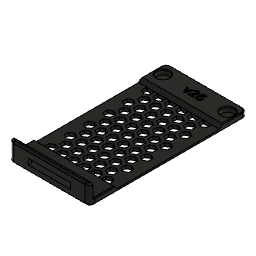
Door_Mount_M1 (Autodesk Fusion 360 design; units mm, degrees)
Autodesk Fusion 360 part; units mm, degrees
note: some values were not read from the file. Set by a fixed rule: which sketch regions a step uses.
(part 1 of 2)
sketch "Skizze1" plane through (0, 0, 0) normal (0, 0, 1) x (1, 0, 0)
  line L0 (22, -48.5) -> (-22, -48.5)
  line L1 (-25, -45.5) -> (-25, 45.5)
  line L2 (-22, 48.5) -> (22, 48.5)
  line L3 (25, 45.5) -> (25, -45.5)
  line L4 (25, -48.5) -> (-25, 48.5) construction
  line L5 (-25, -48.5) -> (25, 48.5) construction
  arc A0 (-22, 48.5) -> (-25, 45.5) centre (-22, 45.5) ccw
  arc A1 (25, 45.5) -> (22, 48.5) centre (22, 45.5) ccw
  arc A2 (22, -48.5) -> (25, -45.5) centre (22, -45.5) ccw
  arc A3 (-25, -45.5) -> (-22, -48.5) centre (-22, -45.5) ccw
  dimension "d356" = 50
  dimension "d357" = 97
  dimension "d358" = 3
  constraint horizontal L0
  constraint perpendicular L0 L1
  constraint parallel L0 L2
  constraint parallel L1 L3
  constraint coincident L4 origin
  constraint coincident L5 origin
  constraint coincident L4.end L1
  constraint coincident L4.end L2
  constraint tangent L1 A0
  constraint tangent L2 A0
  constraint coincident L5.end L2
  constraint coincident L5.end L3
  constraint tangent L2 A1
  constraint tangent L3 A1
  constraint equal A0 A1
  constraint coincident L4.start L3
  constraint coincident L4.start L0
  constraint tangent L3 A2
  constraint tangent L0 A2
  constraint equal A0 A2
  constraint coincident L5.start L0
  constraint coincident L5.start L1
  constraint tangent L0 A3
  constraint tangent L1 A3
  constraint equal A0 A3
  measures "d356" distance of L4.end L5.end
  measures "d357" distance of L5.start L4.end
  measures "d358" radius of A0
extrude "Extrusion1" add sketch "Skizze1" along normal blind 4
sketch "Skizze2" plane through (0, 0, 4) normal (0, 0, 1) x (-1, 0, 0)
  line L0 (24.8284, 46.5) -> (-24.8284, 46.5)
  line L1 (22, 48.5) -> (-22, 48.5)
  arc A0 (-22, 48.5) -> (-25, 45.5) centre (-22, 45.5) ccw
  arc A1 (25, 45.5) -> (22, 48.5) centre (22, 45.5) ccw
  dimension "d416" = 2
  constraint horizontal L0
  constraint coincident L0.end A0
  constraint coincident L0.start A1
  measures "d416" distance of L0 L1
extrude "Extrusion2" add sketch "Skizze2" along normal blind 8
ref_plane "Arbeitsebene1" through (0, 0, 4) normal (0, 0, 1) x (1, 0, 0)
sketch "Skizze3" plane through (0, 0, 4) normal (0, 0, 1) x (1, 0, 0)
  line L0 (-22, -48.5) -> (22, -48.5)
  line L1 (22, -48.5) -> (-22, -48.5)
  line L2 (-13, -46.5) -> (13, -46.5)
  line L3 (13, -46.5) -> (13, -48.5)
  line L4 (13, -48.5) -> (-13, -48.5)
  line L5 (-13, -48.5) -> (-13, -46.5)
  line L6 (-22, 48.5) -> (22, 48.5)
  line L7 (24.8284, -46.5) -> (-24.8284, -46.5)
  dimension "d371" = 26
  dimension "d372" = 13
  constraint horizontal L2
  constraint vertical L3
  constraint horizontal L4
  constraint vertical L5
  constraint coincident L0 L3.end
  constraint coincident L2.start L7
  measures "d371" distance of L3 L5
  measures "d372" distance of origin L5
extrude "Extrusion3" cut sketch "Skizze3" along normal blind 3.5
sketch "Skizze5" plane through (0, 0, 4) normal (0, 0, 1) x (-1, 0, 0)
  line L0 (-25, 45.5) -> (-25, -45.5)
  arc A0 (-25, -45.5) -> (-22, -48.5) centre (-22, -45.5) ccw
  line L1 (-22, -48.5) -> (22, -48.5)
  arc A1 (22, -48.5) -> (25, -45.5) centre (22, -45.5) ccw
  line L2 (25, -45.5) -> (25, 45.5)
  circle A2 centre (20, -41.5) radius 3.75
  circle A3 centre (-20, -41.5) radius 3.75
  line L3 (24.8284, 46.5) -> (13, 46.5)
  arc A4 (-24.8284, 46.5) -> (-25, 45.5) centre (-22, 45.5) ccw
  arc A5 (25, 45.5) -> (24.8284, 46.5) centre (22, 45.5) ccw
  line L4 (13, 46.5) -> (13, 48.5)
  line L5 (13, 48.5) -> (-13, 48.5)
  line L6 (-13, 48.5) -> (-13, 46.5)
  line L7 (-13, 46.5) -> (-24.8284, 46.5)
  dimension "d406" = 7.5
  dimension "d407" = 40
  dimension "d408" = 20
  constraint horizontal A2.centre A3.centre
  constraint equal A2 A3
  measures "d406" diameter of A2
  measures "d407" distance of A2.centre A3.centre
  measures "d408" horizontal distance of origin A2.centre
extrude "Extrusion4" cut sketch "Skizze5" against normal blind 3 contours A2 | A3
sketch "Skizze6" plane through (0, 0, 4) normal (0, 0, 1) x (-1, 0, 0)
  line L0 (24.8284, 46.5) -> (13, 46.5)
  line L1 (13, 46.5) -> (13, 48.5)
  line L2 (13, 48.5) -> (-13, 48.5)
  line L3 (-13, 48.5) -> (-13, 46.5)
  line L4 (-13, 46.5) -> (-24.8284, 46.5)
  line L5 (5.5, -38.5) -> (-5.5, -38.5) construction
  line L6 (-5.5, -38.5) -> (-5.5, -43.5) construction
  line L7 (-5.5, -43.5) -> (5.5, -43.5) construction
  line L8 (5.5, -43.5) -> (5.5, -38.5) construction
  circle A0 centre (20, -41.5) radius 3.75
  circle A1 centre (-20, -41.5) radius 3.75
  arc A2 (-24.8284, 46.5) -> (-25, 45.5) centre (-22, 45.5) ccw
  line L9 (-25, 45.5) -> (-25, -45.5)
  arc A3 (-25, -45.5) -> (-22, -48.5) centre (-22, -45.5) ccw
  line L10 (-22, -48.5) -> (22, -48.5)
  arc A4 (22, -48.5) -> (25, -45.5) centre (22, -45.5) ccw
  line L11 (25, -45.5) -> (25, 45.5)
  arc A5 (25, 45.5) -> (24.8284, 46.5) centre (22, 45.5) ccw
  dimension "d417" = 5
  dimension "d418" = 5
  dimension "d420" = 11
  dimension "d435" = 5
  text T0 "v25" font "Arial" height 5 bold align centre middle in box 11 x 5 at (5.5, -38.5) x (-1, 0) y (0, -1) spacing 1
  constraint vertical origin
  measures "d435" distance of L7 L10
extrude "Extrusion5" cut sketch "Skizze6" against normal blind 0.3 text T0
sketch "Skizze8" plane through (0, 0, 4) normal (0, 0, 1) x (-1, 0, 0)
  line L0 (24.8284, 46.5) -> (13, 46.5)
  line L1 (13, 46.5) -> (13, 48.5)
  line L2 (13, 48.5) -> (-13, 48.5)
  line L3 (-13, 48.5) -> (-13, 46.5)
  line L4 (-13, 46.5) -> (-24.8284, 46.5)
  arc A0 (-24.8284, 46.5) -> (-25, 45.5) centre (-22, 45.5) ccw
  line L5 (-25, 45.5) -> (-25, -45.5)
  arc A1 (-25, -45.5) -> (-22, -48.5) centre (-22, -45.5) ccw
  line L6 (-22, -48.5) -> (22, -48.5)
  arc A2 (22, -48.5) -> (25, -45.5) centre (22, -45.5) ccw
  line L7 (25, -45.5) -> (25, 45.5)
  arc A3 (25, 45.5) -> (24.8284, 46.5) centre (22, 45.5) ccw
  circle A4 centre (-20, -41.5) radius 3.75
  circle A5 centre (20, -41.5) radius 3.75
  line L8 (1.9407, -42.1221) -> (3.3799, -38.5)
  line L9 (3.3799, -38.5) -> (4.2428, -38.5)
  line L10 (4.2428, -38.5) -> (5.7026, -42.1221)
  line L11 (5.7026, -42.1221) -> (4.6965, -42.1221)
  line L12 (4.6965, -42.1221) -> (4.0143, -40.2735)
  line L13 (4.0143, -40.2735) -> (3.8165, -39.6562)
  spline S0 degree 3 poles (3.8165, -39.6562) (3.7947, -39.7212) (3.7602, -39.8241) (3.7291, -39.9282) (3.7176, -39.9666) knots 0 0 0 0 0.020546 0.032577 0.032577 0.032577 0.032577
  spline S1 degree 3 poles (3.7176, -39.9666) (3.7014, -40.0178) (3.6688, -40.1207) (3.6332, -40.2225) (3.6153, -40.2735) knots 0 0 0 0 0.016125 0.032358 0.032358 0.032358 0.032358
  line L14 (3.6153, -40.2735) -> (2.9263, -42.1221)
  line L15 (2.9263, -42.1221) -> (1.9407, -42.1221)
  line L16 (-1.678, -39.3902) -> (-1.678, -38.5)
  line L17 (-1.678, -38.5) -> (1.6814, -38.5)
  spline S2 degree 3 poles (1.6814, -38.5) (1.6537, -38.6668) (1.5977, -39.0038) (1.4358, -39.3047) (1.354, -39.4567) knots 0 0 0 0 0.050353 0.101733 0.101733 0.101733 0.101733
  spline S3 degree 3 poles (0.2763, -40.6555) (0.0973, -40.8199) (-0.1834, -41.0777) (-0.4293, -41.3686) (-0.5184, -41.4741) knots 0 0 0 0 0.072782 0.114179 0.114179 0.114179 0.114179
  spline S4 degree 3 poles (-0.5184, -41.4741) (-0.5761, -41.5697) (-0.6853, -41.7511) (-0.7063, -41.9614) (-0.7162, -42.0607) knots 0 0 0 0 0.033023 0.0626 0.0626 0.0626 0.0626
  line L18 (25, -33.5) -> (-25, -33.5)
  line L19 (25, 33.5) -> (-25, 33.5)
  line L20 (-13, 48.5) -> (13, 48.5)
  line L21 (13, 48.5) -> (-13, 48.5)
  line L22 (22, 48.5) -> (-22, 48.5)
  line L23 (-22, 48.5) -> (22, 48.5)
  spline S5 degree 3 poles (1.5689, -42.0402) (1.5336, -42.2784) (1.469, -42.7135) (1.1692, -43.0319) (1.0334, -43.176) knots 0 0 0 0 0.070212 0.128259 0.128259 0.128259 0.128259
  spline S6 degree 3 poles (1.0334, -43.176) (0.8691, -43.2764) (0.5241, -43.4872) (0.1197, -43.509) (-0.0921, -43.5205) knots 0 0 0 0 0.056857 0.119356 0.119356 0.119356 0.119356
  spline S7 degree 3 poles (-0.0921, -43.5205) (-0.3201, -43.5088) (-0.7475, -43.4868) (-1.0936, -43.2377) (-1.2551, -43.1214) knots 0 0 0 0 0.06683 0.125293 0.125293 0.125293 0.125293
  spline S8 degree 3 poles (-1.678, -42.1289) (-1.6731, -42.0181) (-1.6634, -41.798) (-1.5923, -41.5895) (-1.557, -41.486) knots 0 0 0 0 0.033094 0.065719 0.065719 0.065719 0.065719
  spline S9 degree 3 poles (-1.557, -41.486) (-1.5082, -41.3799) (-1.4037, -41.1528) (-1.2534, -40.9529) (-1.1733, -40.8465) knots 0 0 0 0 0.034948 0.074768 0.074768 0.074768 0.074768
  spline S10 degree 3 poles (0.4093, -42.545) (0.4624, -42.4673) (0.5854, -42.2873) (0.6036, -42.0688) (0.6139, -41.9447) knots 0 0 0 0 0.027816 0.064377 0.064377 0.064377 0.064377
  spline S11 degree 3 poles (-1.2551, -43.1214) (-1.3785, -42.9797) (-1.6266, -42.6947) (-1.6608, -42.3182) (-1.678, -42.1289) knots 0 0 0 0 0.054863 0.110365 0.110365 0.110365 0.110365
  spline S12 degree 3 poles (-1.1733, -40.8465) (-1.0933, -40.7552) (-0.8965, -40.5305) (-0.6764, -40.3286) (-0.5457, -40.2087) knots 0 0 0 0 0.036404 0.089534 0.089534 0.089534 0.089534
  spline S13 degree 3 poles (-0.5457, -40.2087) (-0.4207, -40.0948) (-0.2242, -39.9158) (-0.0386, -39.7255) (0.029, -39.6562) knots 0 0 0 0 0.050705 0.079736 0.079736 0.079736 0.079736
  spline S14 degree 3 poles (0.029, -39.6562) (0.0667, -39.6122) (0.1387, -39.5283) (0.1973, -39.4347) (0.2251, -39.3902) knots 0 0 0 0 0.017365 0.033092 0.033092 0.033092 0.033092
  line L24 (0.2251, -39.3902) -> (-1.678, -39.3902)
  spline S15 degree 3 poles (1.354, -39.4567) (1.2231, -39.6357) (0.9046, -40.0712) (0.5091, -40.439) (0.2763, -40.6555) knots 0 0 0 0 0.066412 0.161523 0.161523 0.161523 0.161523
  spline S16 degree 3 poles (-0.7162, -42.0607) (-0.7115, -42.1588) (-0.7028, -42.3409) (-0.5942, -42.4864) (-0.544, -42.5535) knots 0 0 0 0 0.028676 0.053274 0.053274 0.053274 0.053274
  spline S17 degree 3 poles (-0.544, -42.5535) (-0.4783, -42.6037) (-0.3384, -42.7107) (-0.1619, -42.7205) (-0.0682, -42.7258) knots 0 0 0 0 0.024236 0.051648 0.051648 0.051648 0.051648
  spline S18 degree 3 poles (-0.0682, -42.7258) (0.0251, -42.7198) (0.2033, -42.7084) (0.3429, -42.5977) (0.4093, -42.545) knots 0 0 0 0 0.02732 0.052153 0.052153 0.052153 0.052153
  line L25 (0.6139, -41.9447) -> (1.5689, -42.0402)
  line L26 (-2.3397, -39.7858) -> (-3.2947, -39.8847)
  line L27 (-3.2333, -40.7169) -> (-2.4557, -40.8295)
  line L28 (-2.4557, -40.8295) -> (-2.9468, -43.4318)
  line L29 (-2.9468, -43.4318) -> (-5.4809, -43.4318)
  spline S19 degree 3 poles (-3.9905, -38.4147) (-3.7745, -38.4268) (-3.3639, -38.4497) (-3.0231, -38.6781) (-2.8615, -38.7865) knots 0 0 0 0 0.063525 0.120818 0.120818 0.120818 0.120818
  spline S20 degree 3 poles (-2.8615, -38.7865) (-2.7303, -38.9238) (-2.4604, -39.2062) (-2.3807, -39.5891) (-2.3397, -39.7858) knots 0 0 0 0 0.055809 0.114768 0.114768 0.114768 0.114768
  spline S21 degree 3 poles (-3.2947, -39.8847) (-3.3134, -39.7839) (-3.3491, -39.5912) (-3.4762, -39.4424) (-3.5368, -39.3714) knots 0 0 0 0 0.030142 0.057653 0.057653 0.057653 0.057653
  spline S22 degree 3 poles (-3.5368, -39.3714) (-3.6058, -39.3162) (-3.7419, -39.2073) (-3.9152, -39.1905) (-4.0007, -39.1821) knots 0 0 0 0 0.025896 0.051072 0.051072 0.051072 0.051072
  spline S23 degree 3 poles (-4.0007, -39.1821) (-4.0975, -39.193) (-4.2949, -39.2153) (-4.4367, -39.3549) (-4.5089, -39.426) knots 0 0 0 0 0.028374 0.057844 0.057844 0.057844 0.057844
  spline S24 degree 3 poles (-4.5089, -39.426) (-4.5693, -39.5253) (-4.706, -39.7497) (-4.713, -40.0138) (-4.7169, -40.161) knots 0 0 0 0 0.03432 0.077565 0.077565 0.077565 0.077565
  spline S25 degree 3 poles (-4.7169, -40.161) (-4.7127, -40.2994) (-4.7052, -40.5493) (-4.5706, -40.7584) (-4.5106, -40.8516) knots 0 0 0 0 0.040617 0.073292 0.073292 0.073292 0.073292
  spline S26 degree 3 poles (-4.5106, -40.8516) (-4.4356, -40.9188) (-4.2826, -41.0557) (-4.0778, -41.073) (-3.9734, -41.0819) knots 0 0 0 0 0.02936 0.059879 0.059879 0.059879 0.059879
  spline S27 degree 3 poles (-3.9734, -41.0819) (-3.837, -41.0639) (-3.5501, -41.0261) (-3.3423, -40.8233) (-3.2333, -40.7169) knots 0 0 0 0 0.040186 0.084518 0.084518 0.084518 0.084518
  line L30 (-5.4809, -43.4318) -> (-5.4809, -42.5348)
  line L31 (-5.4809, -42.5348) -> (-3.6733, -42.5348)
  line L32 (-3.6733, -42.5348) -> (-3.5232, -41.6855)
  spline S28 degree 3 poles (-3.5232, -41.6855) (-3.6296, -41.7323) (-3.8385, -41.8241) (-4.0663, -41.8387) (-4.178, -41.8458) knots 0 0 0 0 0.03456 0.067885 0.067885 0.067885 0.067885
  spline S29 degree 3 poles (-4.178, -41.8458) (-4.3827, -41.8264) (-4.7926, -41.7874) (-5.1035, -41.5173) (-5.2592, -41.382) knots 0 0 0 0 0.060049 0.120305 0.120305 0.120305 0.120305
  spline S30 degree 3 poles (-5.2592, -41.382) (-5.3885, -41.2113) (-5.6577, -40.8558) (-5.6872, -40.4099) (-5.7026, -40.178) knots 0 0 0 0 0.062815 0.130829 0.130829 0.130829 0.130829
  spline S31 degree 3 poles (-5.7026, -40.178) (-5.6881, -39.9783) (-5.6592, -39.5816) (-5.4489, -39.2441) (-5.3445, -39.0764) knots 0 0 0 0 0.059089 0.1174 0.1174 0.1174 0.1174
  spline S32 degree 3 poles (-5.3445, -39.0764) (-5.164, -38.8834) (-4.7972, -38.4914) (-4.2621, -38.4406) (-3.9905, -38.4147) knots 0 0 0 0 0.076512 0.155431 0.155431 0.155431 0.155431
  dimension "d436" = 15
  dimension "d437" = 15
  constraint coincident L7 L18.start
  constraint coincident L5 L18.end
  constraint perpendicular L5 L18
  constraint coincident L7 L19.start
  constraint coincident L5 L19.end
  constraint perpendicular L5 L19
  measures "d436" distance of L6 L18
  measures "d437" distance of L19 L23
extrude "Extrusion6" cut sketch "Skizze8" against normal blind 2 contours L5 L7 L18 L19
chamfer "Fase1" distance 1 angle 45 11 edges at (0, -48.5, 0) (-24.1213, -47.6213, 0) (-25, 0, 0) (-24.1213, 47.6213, 0) (0, 48.5, 0) (24.1213, 47.6213, 0) (25, 0, 0) (24.1213, -47.6213, 0) (0, -48.5, 12) (-23.7321, -47.9495, 12) (23.7321, -47.9495, 12)
chamfer "Fase1" distance 0.5 angle 45 11 edges at (-16.5038, 40.1439, 4) (23.4962, 40.1439, 4) (25, -39.5, 4) (24.9568, -46.0073, 4) (25, 39.5, 4) (24.1213, 47.6213, 4) (0, 48.5, 4) (-24.1213, 47.6213, 4) (-25, 39.5, 4) (-24.9568, -46.0073, 4) (-25, -39.5, 4)
chamfer "Fase1" distance 2 angle 45 2 edges at (0, 33.5, 2) (0, -33.5, 2)
sketch "Skizze9" plane through (0, 0, 2) normal (0, 0, 1) x (-1, 0, 0)
  line L0 (25, -31.5) -> (25, 31.5)
  line L1 (-25, 31.5) -> (-25, -31.5)
  line L2 (-2.5, -1.4434) -> (0, -2.8868)
  line L3 (0, -2.8868) -> (2.5, -1.4434)
  line L4 (2.5, -1.4434) -> (2.5, 1.4434)
  line L5 (2.5, 1.4434) -> (0, 2.8868)
  line L6 (0, 2.8868) -> (-2.5, 1.4434)
  line L7 (-2.5, 1.4434) -> (-2.5, -1.4434)
  line L8 (-6, 4.6188) -> (-3.5, 3.1754)
  line L9 (-3.5, 3.1754) -> (-1, 4.6188)
  line L10 (-1, 4.6188) -> (-1, 7.5056)
  line L11 (-1, 7.5056) -> (-3.5, 8.9489)
  line L12 (-3.5, 8.9489) -> (-6, 7.5056)
  line L13 (-6, 7.5056) -> (-6, 4.6188)
  line L14 (0, 2.8868) -> (-1, 4.6188) construction
  line L15 (-7, 2.8868) -> (-9.5, 1.4434)
  line L16 (-9.5, 1.4434) -> (-9.5, -1.4434)
  line L17 (-9.5, -1.4434) -> (-7, -2.8868)
  line L18 (-7, -2.8868) -> (-4.5, -1.4434)
  line L19 (-4.5, -1.4434) -> (-4.5, 1.4434)
  line L20 (-4.5, 1.4434) -> (-7, 2.8868)
  line L21 (-3.5, 3.1754) -> (-4.5, 1.4434) construction
  line L22 (1, 7.5056) -> (1, 4.6188)
  line L23 (1, 4.6188) -> (3.5, 3.1754)
  line L24 (3.5, 3.1754) -> (6, 4.6188)
  line L25 (6, 4.6188) -> (6, 7.5056)
  line L26 (6, 7.5056) -> (3.5, 8.9489)
  line L27 (3.5, 8.9489) -> (1, 7.5056)
  line L28 (2.5, 1.4434) -> (3.5, 3.1754) construction
  line L29 (-24.5, -32.8246) -> (-22, -31.3812)
  line L30 (-22, -31.3812) -> (-22, -28.4944)
  line L31 (-22, -28.4944) -> (-24.5, -27.0511)
  line L32 (-24.5, -27.0511) -> (-27, -28.4944)
  line L33 (-27, -28.4944) -> (-27, -31.3812)
  line L34 (-27, -31.3812) -> (-24.5, -32.8246)
  line L35 (-25.5, -34.5566) -> (-28, -33.1132)
  line L36 (-25.5, -37.4434) -> (-25.5, -34.5566)
  line L37 (-28, -38.8868) -> (-25.5, -37.4434)
  line L38 (-30.5, -37.4434) -> (-28, -38.8868)
  line L39 (-30.5, -34.5566) -> (-30.5, -37.4434)
  line L40 (-28, -33.1132) -> (-30.5, -34.5566)
  line L41 (-31.5, -32.8246) -> (-29, -31.3812)
  line L42 (-29, -31.3812) -> (-29, -28.4944)
  line L43 (-29, -28.4944) -> (-31.5, -27.0511)
  line L44 (-34, -31.3812) -> (-31.5, -32.8246)
  line L45 (-31.5, -27.0511) -> (-34, -28.4944)
  line L46 (-34, -28.4944) -> (-34, -31.3812)
  line L47 (-35, -33.1132) -> (-37.5, -34.5566)
  line L48 (-32.5, -34.5566) -> (-35, -33.1132)
  line L49 (-32.5, -37.4434) -> (-32.5, -34.5566)
  line L50 (-35, -38.8868) -> (-32.5, -37.4434)
  line L51 (-37.5, -37.4434) -> (-35, -38.8868)
  line L52 (-37.5, -34.5566) -> (-37.5, -37.4434)
  line L53 (-10.5, -32.8246) -> (-8, -31.3812)
  line L54 (-8, -31.3812) -> (-8, -28.4944)
  line L55 (-8, -28.4944) -> (-10.5, -27.0511)
  line L56 (-10.5, -27.0511) -> (-13, -28.4944)
  line L57 (-13, -28.4944) -> (-13, -31.3812)
  line L58 (-13, -31.3812) -> (-10.5, -32.8246)
  line L59 (-11.5, -34.5566) -> (-14, -33.1132)
  line L60 (-11.5, -37.4434) -> (-11.5, -34.5566)
  line L61 (-14, -38.8868) -> (-11.5, -37.4434)
  line L62 (-16.5, -37.4434) -> (-14, -38.8868)
  line L63 (-16.5, -34.5566) -> (-16.5, -37.4434)
  line L64 (-14, -33.1132) -> (-16.5, -34.5566)
  line L65 (-17.5, -32.8246) -> (-15, -31.3812)
  line L66 (-15, -31.3812) -> (-15, -28.4944)
  line L67 (-15, -28.4944) -> (-17.5, -27.0511)
  line L68 (-20, -31.3812) -> (-17.5, -32.8246)
  line L69 (-17.5, -27.0511) -> (-20, -28.4944)
  line L70 (-20, -28.4944) -> (-20, -31.3812)
  line L71 (-21, -33.1132) -> (-23.5, -34.5566)
  line L72 (-18.5, -34.5566) -> (-21, -33.1132)
  line L73 (-18.5, -37.4434) -> (-18.5, -34.5566)
  line L74 (-21, -38.8868) -> (-18.5, -37.4434)
  line L75 (-23.5, -37.4434) -> (-21, -38.8868)
  line L76 (-23.5, -34.5566) -> (-23.5, -37.4434)
  line L77 (3.5, -32.8246) -> (6, -31.3812)
  line L78 (6, -31.3812) -> (6, -28.4944)
  line L79 (6, -28.4944) -> (3.5, -27.0511)
  line L80 (3.5, -27.0511) -> (1, -28.4944)
  line L81 (1, -28.4944) -> (1, -31.3812)
  line L82 (1, -31.3812) -> (3.5, -32.8246)
  line L83 (2.5, -34.5566) -> (0, -33.1132)
  line L84 (2.5, -37.4434) -> (2.5, -34.5566)
  line L85 (0, -38.8868) -> (2.5, -37.4434)
  line L86 (-2.5, -37.4434) -> (0, -38.8868)
  line L87 (-2.5, -34.5566) -> (-2.5, -37.4434)
  line L88 (0, -33.1132) -> (-2.5, -34.5566)
  line L89 (-3.5, -32.8246) -> (-1, -31.3812)
  line L90 (-1, -31.3812) -> (-1, -28.4944)
  line L91 (-1, -28.4944) -> (-3.5, -27.0511)
  line L92 (-6, -31.3812) -> (-3.5, -32.8246)
  line L93 (-3.5, -27.0511) -> (-6, -28.4944)
  line L94 (-6, -28.4944) -> (-6, -31.3812)
  line L95 (-7, -33.1132) -> (-9.5, -34.5566)
  line L96 (-4.5, -34.5566) -> (-7, -33.1132)
  line L97 (-4.5, -37.4434) -> (-4.5, -34.5566)
  line L98 (-7, -38.8868) -> (-4.5, -37.4434)
  line L99 (-9.5, -37.4434) -> (-7, -38.8868)
  line L100 (-9.5, -34.5566) -> (-9.5, -37.4434)
  line L101 (17.5, -32.8246) -> (20, -31.3812)
  line L102 (20, -31.3812) -> (20, -28.4944)
  line L103 (20, -28.4944) -> (17.5, -27.0511)
  line L104 (17.5, -27.0511) -> (15, -28.4944)
  line L105 (15, -28.4944) -> (15, -31.3812)
  line L106 (15, -31.3812) -> (17.5, -32.8246)
  line L107 (16.5, -34.5566) -> (14, -33.1132)
  line L108 (16.5, -37.4434) -> (16.5, -34.5566)
  line L109 (14, -38.8868) -> (16.5, -37.4434)
  line L110 (11.5, -37.4434) -> (14, -38.8868)
  line L111 (11.5, -34.5566) -> (11.5, -37.4434)
  line L112 (14, -33.1132) -> (11.5, -34.5566)
  line L113 (10.5, -32.8246) -> (13, -31.3812)
  line L114 (13, -31.3812) -> (13, -28.4944)
  line L115 (13, -28.4944) -> (10.5, -27.0511)
  line L116 (8, -31.3812) -> (10.5, -32.8246)
  line L117 (10.5, -27.0511) -> (8, -28.4944)
  line L118 (8, -28.4944) -> (8, -31.3812)
  line L119 (7, -33.1132) -> (4.5, -34.5566)
  line L120 (9.5, -34.5566) -> (7, -33.1132)
  line L121 (9.5, -37.4434) -> (9.5, -34.5566)
  line L122 (7, -38.8868) -> (9.5, -37.4434)
  line L123 (4.5, -37.4434) -> (7, -38.8868)
  line L124 (4.5, -34.5566) -> (4.5, -37.4434)
  line L125 (31.5, -32.8246) -> (34, -31.3812)
  line L126 (34, -31.3812) -> (34, -28.4944)
  line L127 (34, -28.4944) -> (31.5, -27.0511)
  line L128 (31.5, -27.0511) -> (29, -28.4944)
  line L129 (29, -28.4944) -> (29, -31.3812)
  line L130 (29, -31.3812) -> (31.5, -32.8246)
  line L131 (30.5, -34.5566) -> (28, -33.1132)
  line L132 (30.5, -37.4434) -> (30.5, -34.5566)
  line L133 (28, -38.8868) -> (30.5, -37.4434)
  line L134 (25.5, -37.4434) -> (28, -38.8868)
  line L135 (25.5, -34.5566) -> (25.5, -37.4434)
  line L136 (28, -33.1132) -> (25.5, -34.5566)
  line L137 (24.5, -32.8246) -> (27, -31.3812)
  line L138 (27, -31.3812) -> (27, -28.4944)
  line L139 (27, -28.4944) -> (24.5, -27.0511)
  line L140 (22, -31.3812) -> (24.5, -32.8246)
  line L141 (24.5, -27.0511) -> (22, -28.4944)
  line L142 (22, -28.4944) -> (22, -31.3812)
  line L143 (21, -33.1132) -> (18.5, -34.5566)
  line L144 (23.5, -34.5566) -> (21, -33.1132)
  line L145 (23.5, -37.4434) -> (23.5, -34.5566)
  line L146 (21, -38.8868) -> (23.5, -37.4434)
  line L147 (18.5, -37.4434) -> (21, -38.8868)
  line L148 (18.5, -34.5566) -> (18.5, -37.4434)
  line L149 (-24.5, -20.8246) -> (-22, -19.3812)
  line L150 (-22, -19.3812) -> (-22, -16.4944)
  line L151 (-22, -16.4944) -> (-24.5, -15.0511)
  line L152 (-24.5, -15.0511) -> (-27, -16.4944)
  line L153 (-27, -16.4944) -> (-27, -19.3812)
  line L154 (-27, -19.3812) -> (-24.5, -20.8246)
  line L155 (-25.5, -22.5566) -> (-28, -21.1132)
  line L156 (-25.5, -25.4434) -> (-25.5, -22.5566)
  line L157 (-28, -26.8868) -> (-25.5, -25.4434)
  line L158 (-30.5, -25.4434) -> (-28, -26.8868)
  line L159 (-30.5, -22.5566) -> (-30.5, -25.4434)
  line L160 (-28, -21.1132) -> (-30.5, -22.5566)
  line L161 (-31.5, -20.8246) -> (-29, -19.3812)
  line L162 (-29, -19.3812) -> (-29, -16.4944)
  line L163 (-29, -16.4944) -> (-31.5, -15.0511)
  line L164 (-34, -19.3812) -> (-31.5, -20.8246)
  line L165 (-31.5, -15.0511) -> (-34, -16.4944)
  line L166 (-34, -16.4944) -> (-34, -19.3812)
  line L167 (-35, -21.1132) -> (-37.5, -22.5566)
  line L168 (-32.5, -22.5566) -> (-35, -21.1132)
  line L169 (-32.5, -25.4434) -> (-32.5, -22.5566)
  line L170 (-35, -26.8868) -> (-32.5, -25.4434)
  line L171 (-37.5, -25.4434) -> (-35, -26.8868)
  line L172 (-37.5, -22.5566) -> (-37.5, -25.4434)
  line L173 (-10.5, -20.8246) -> (-8, -19.3812)
  line L174 (-8, -19.3812) -> (-8, -16.4944)
  line L175 (-8, -16.4944) -> (-10.5, -15.0511)
  line L176 (-10.5, -15.0511) -> (-13, -16.4944)
  line L177 (-13, -16.4944) -> (-13, -19.3812)
  line L178 (-13, -19.3812) -> (-10.5, -20.8246)
  line L179 (-11.5, -22.5566) -> (-14, -21.1132)
  line L180 (-11.5, -25.4434) -> (-11.5, -22.5566)
  line L181 (-14, -26.8868) -> (-11.5, -25.4434)
  line L182 (-16.5, -25.4434) -> (-14, -26.8868)
  line L183 (-16.5, -22.5566) -> (-16.5, -25.4434)
  line L184 (-14, -21.1132) -> (-16.5, -22.5566)
  line L185 (-17.5, -20.8246) -> (-15, -19.3812)
  line L186 (-15, -19.3812) -> (-15, -16.4944)
  line L187 (-15, -16.4944) -> (-17.5, -15.0511)
  line L188 (-20, -19.3812) -> (-17.5, -20.8246)
  line L189 (-17.5, -15.0511) -> (-20, -16.4944)
  line L190 (-20, -16.4944) -> (-20, -19.3812)
  line L191 (-21, -21.1132) -> (-23.5, -22.5566)
  line L192 (-18.5, -22.5566) -> (-21, -21.1132)
  line L193 (-18.5, -25.4434) -> (-18.5, -22.5566)
  line L194 (-21, -26.8868) -> (-18.5, -25.4434)
  line L195 (-23.5, -25.4434) -> (-21, -26.8868)
  line L196 (-23.5, -22.5566) -> (-23.5, -25.4434)
  line L197 (3.5, -20.8246) -> (6, -19.3812)
  line L198 (6, -19.3812) -> (6, -16.4944)
  line L199 (6, -16.4944) -> (3.5, -15.0511)
  line L200 (3.5, -15.0511) -> (1, -16.4944)
  line L201 (1, -16.4944) -> (1, -19.3812)
  line L202 (1, -19.3812) -> (3.5, -20.8246)
  line L203 (2.5, -22.5566) -> (0, -21.1132)
  line L204 (2.5, -25.4434) -> (2.5, -22.5566)
  line L205 (0, -26.8868) -> (2.5, -25.4434)
  line L206 (-2.5, -25.4434) -> (0, -26.8868)
  line L207 (-2.5, -22.5566) -> (-2.5, -25.4434)
  line L208 (0, -21.1132) -> (-2.5, -22.5566)
  line L209 (-3.5, -20.8246) -> (-1, -19.3812)
  line L210 (-1, -19.3812) -> (-1, -16.4944)
  line L211 (-1, -16.4944) -> (-3.5, -15.0511)
  line L212 (-6, -19.3812) -> (-3.5, -20.8246)
  line L213 (-3.5, -15.0511) -> (-6, -16.4944)
  line L214 (-6, -16.4944) -> (-6, -19.3812)
  line L215 (-7, -21.1132) -> (-9.5, -22.5566)
  line L216 (-4.5, -22.5566) -> (-7, -21.1132)
  line L217 (-4.5, -25.4434) -> (-4.5, -22.5566)
  line L218 (-7, -26.8868) -> (-4.5, -25.4434)
  line L219 (-9.5, -25.4434) -> (-7, -26.8868)
  line L220 (-9.5, -22.5566) -> (-9.5, -25.4434)
  line L221 (17.5, -20.8246) -> (20, -19.3812)
  line L222 (20, -19.3812) -> (20, -16.4944)
  line L223 (20, -16.4944) -> (17.5, -15.0511)
  line L224 (17.5, -15.0511) -> (15, -16.4944)
  line L225 (15, -16.4944) -> (15, -19.3812)
  line L226 (15, -19.3812) -> (17.5, -20.8246)
  line L227 (16.5, -22.5566) -> (14, -21.1132)
  line L228 (16.5, -25.4434) -> (16.5, -22.5566)
  line L229 (14, -26.8868) -> (16.5, -25.4434)
  line L230 (11.5, -25.4434) -> (14, -26.8868)
  line L231 (11.5, -22.5566) -> (11.5, -25.4434)
  line L232 (14, -21.1132) -> (11.5, -22.5566)
  line L233 (10.5, -20.8246) -> (13, -19.3812)
  line L234 (13, -19.3812) -> (13, -16.4944)
  line L235 (13, -16.4944) -> (10.5, -15.0511)
  line L236 (8, -19.3812) -> (10.5, -20.8246)
  line L237 (10.5, -15.0511) -> (8, -16.4944)
  line L238 (8, -16.4944) -> (8, -19.3812)
  line L239 (7, -21.1132) -> (4.5, -22.5566)
  line L240 (9.5, -22.5566) -> (7, -21.1132)
  line L241 (9.5, -25.4434) -> (9.5, -22.5566)
  line L242 (7, -26.8868) -> (9.5, -25.4434)
  line L243 (4.5, -25.4434) -> (7, -26.8868)
  line L244 (4.5, -22.5566) -> (4.5, -25.4434)
  line L245 (31.5, -20.8246) -> (34, -19.3812)
  line L246 (34, -19.3812) -> (34, -16.4944)
  line L247 (34, -16.4944) -> (31.5, -15.0511)
  line L248 (31.5, -15.0511) -> (29, -16.4944)
  line L249 (29, -16.4944) -> (29, -19.3812)
  line L250 (29, -19.3812) -> (31.5, -20.8246)
  line L251 (30.5, -22.5566) -> (28, -21.1132)
  line L252 (30.5, -25.4434) -> (30.5, -22.5566)
  line L253 (28, -26.8868) -> (30.5, -25.4434)
  line L254 (25.5, -25.4434) -> (28, -26.8868)
  line L255 (25.5, -22.5566) -> (25.5, -25.4434)
  line L256 (28, -21.1132) -> (25.5, -22.5566)
  line L257 (24.5, -20.8246) -> (27, -19.3812)
  line L258 (27, -19.3812) -> (27, -16.4944)
  line L259 (27, -16.4944) -> (24.5, -15.0511)
  line L260 (22, -19.3812) -> (24.5, -20.8246)
  line L261 (24.5, -15.0511) -> (22, -16.4944)
  line L262 (22, -16.4944) -> (22, -19.3812)
  line L263 (21, -21.1132) -> (18.5, -22.5566)
  line L264 (23.5, -22.5566) -> (21, -21.1132)
  line L265 (23.5, -25.4434) -> (23.5, -22.5566)
  line L266 (21, -26.8868) -> (23.5, -25.4434)
  line L267 (18.5, -25.4434) -> (21, -26.8868)
  line L268 (18.5, -22.5566) -> (18.5, -25.4434)
  line L269 (-24.5, -8.8246) -> (-22, -7.3812)
  line L270 (-22, -7.3812) -> (-22, -4.4944)
  line L271 (-22, -4.4944) -> (-24.5, -3.0511)
  line L272 (-24.5, -3.0511) -> (-27, -4.4944)
  line L273 (-27, -4.4944) -> (-27, -7.3812)
  line L274 (-27, -7.3812) -> (-24.5, -8.8246)
  line L275 (-25.5, -10.5566) -> (-28, -9.1132)
  line L276 (-25.5, -13.4434) -> (-25.5, -10.5566)
  line L277 (-28, -14.8868) -> (-25.5, -13.4434)
  line L278 (-30.5, -13.4434) -> (-28, -14.8868)
  line L279 (-30.5, -10.5566) -> (-30.5, -13.4434)
  line L280 (-28, -9.1132) -> (-30.5, -10.5566)
  line L281 (-31.5, -8.8246) -> (-29, -7.3812)
  line L282 (-29, -7.3812) -> (-29, -4.4944)
  line L283 (-29, -4.4944) -> (-31.5, -3.0511)
  line L284 (-34, -7.3812) -> (-31.5, -8.8246)
  line L285 (-31.5, -3.0511) -> (-34, -4.4944)
  line L286 (-34, -4.4944) -> (-34, -7.3812)
  line L287 (-35, -9.1132) -> (-37.5, -10.5566)
  line L288 (-32.5, -10.5566) -> (-35, -9.1132)
  line L289 (-32.5, -13.4434) -> (-32.5, -10.5566)
  line L290 (-35, -14.8868) -> (-32.5, -13.4434)
  line L291 (-37.5, -13.4434) -> (-35, -14.8868)
  line L292 (-37.5, -10.5566) -> (-37.5, -13.4434)
  line L293 (-10.5, -8.8246) -> (-8, -7.3812)
  line L294 (-8, -7.3812) -> (-8, -4.4944)
  line L295 (-8, -4.4944) -> (-10.5, -3.0511)
  line L296 (-10.5, -3.0511) -> (-13, -4.4944)
  line L297 (-13, -4.4944) -> (-13, -7.3812)
  line L298 (-13, -7.3812) -> (-10.5, -8.8246)
  line L299 (-11.5, -10.5566) -> (-14, -9.1132)
  line L300 (-11.5, -13.4434) -> (-11.5, -10.5566)
  line L301 (-14, -14.8868) -> (-11.5, -13.4434)
  line L302 (-16.5, -13.4434) -> (-14, -14.8868)
  line L303 (-16.5, -10.5566) -> (-16.5, -13.4434)
  line L304 (-14, -9.1132) -> (-16.5, -10.5566)
  line L305 (-17.5, -8.8246) -> (-15, -7.3812)
  line L306 (-15, -7.3812) -> (-15, -4.4944)
  line L307 (-15, -4.4944) -> (-17.5, -3.0511)
  line L308 (-20, -7.3812) -> (-17.5, -8.8246)
  line L309 (-17.5, -3.0511) -> (-20, -4.4944)
  line L310 (-20, -4.4944) -> (-20, -7.3812)
  line L311 (-21, -9.1132) -> (-23.5, -10.5566)
  line L312 (-18.5, -10.5566) -> (-21, -9.1132)
  line L313 (-18.5, -13.4434) -> (-18.5, -10.5566)
  line L314 (-21, -14.8868) -> (-18.5, -13.4434)
  line L315 (-23.5, -13.4434) -> (-21, -14.8868)
  line L316 (-23.5, -10.5566) -> (-23.5, -13.4434)
  line L317 (3.5, -8.8246) -> (6, -7.3812)
  line L318 (6, -7.3812) -> (6, -4.4944)
  line L319 (6, -4.4944) -> (3.5, -3.0511)
  line L320 (3.5, -3.0511) -> (1, -4.4944)
  line L321 (1, -4.4944) -> (1, -7.3812)
  line L322 (1, -7.3812) -> (3.5, -8.8246)
  line L323 (2.5, -10.5566) -> (0, -9.1132)
  line L324 (2.5, -13.4434) -> (2.5, -10.5566)
  line L325 (0, -14.8868) -> (2.5, -13.4434)
  line L326 (-2.5, -13.4434) -> (0, -14.8868)
  line L327 (-2.5, -10.5566) -> (-2.5, -13.4434)
  line L328 (0, -9.1132) -> (-2.5, -10.5566)
  line L329 (-3.5, -8.8246) -> (-1, -7.3812)
  line L330 (-1, -7.3812) -> (-1, -4.4944)
  line L331 (-1, -4.4944) -> (-3.5, -3.0511)
  line L332 (-6, -7.3812) -> (-3.5, -8.8246)
  line L333 (-3.5, -3.0511) -> (-6, -4.4944)
  line L334 (-6, -4.4944) -> (-6, -7.3812)
  line L335 (-7, -9.1132) -> (-9.5, -10.5566)
  line L336 (-4.5, -10.5566) -> (-7, -9.1132)
  line L337 (-4.5, -13.4434) -> (-4.5, -10.5566)
  line L338 (-7, -14.8868) -> (-4.5, -13.4434)
  line L339 (-9.5, -13.4434) -> (-7, -14.8868)
  line L340 (-9.5, -10.5566) -> (-9.5, -13.4434)
  line L341 (17.5, -8.8246) -> (20, -7.3812)
  line L342 (20, -7.3812) -> (20, -4.4944)
  line L343 (20, -4.4944) -> (17.5, -3.0511)
  line L344 (17.5, -3.0511) -> (15, -4.4944)
  line L345 (15, -4.4944) -> (15, -7.3812)
  line L346 (15, -7.3812) -> (17.5, -8.8246)
  line L347 (16.5, -10.5566) -> (14, -9.1132)
  line L348 (16.5, -13.4434) -> (16.5, -10.5566)
  line L349 (14, -14.8868) -> (16.5, -13.4434)
  line L350 (11.5, -13.4434) -> (14, -14.8868)
  line L351 (11.5, -10.5566) -> (11.5, -13.4434)
  line L352 (14, -9.1132) -> (11.5, -10.5566)
  line L353 (10.5, -8.8246) -> (13, -7.3812)
  line L354 (13, -7.3812) -> (13, -4.4944)
  line L355 (13, -4.4944) -> (10.5, -3.0511)
  line L356 (8, -7.3812) -> (10.5, -8.8246)
  line L357 (10.5, -3.0511) -> (8, -4.4944)
  line L358 (8, -4.4944) -> (8, -7.3812)
  line L359 (7, -9.1132) -> (4.5, -10.5566)
  line L360 (9.5, -10.5566) -> (7, -9.1132)
  line L361 (9.5, -13.4434) -> (9.5, -10.5566)
  line L362 (7, -14.8868) -> (9.5, -13.4434)
  line L363 (4.5, -13.4434) -> (7, -14.8868)
  line L364 (4.5, -10.5566) -> (4.5, -13.4434)
  line L365 (31.5, -8.8246) -> (34, -7.3812)
  line L366 (34, -7.3812) -> (34, -4.4944)
  line L367 (34, -4.4944) -> (31.5, -3.0511)
  line L368 (31.5, -3.0511) -> (29, -4.4944)
  line L369 (29, -4.4944) -> (29, -7.3812)
  line L370 (29, -7.3812) -> (31.5, -8.8246)
  line L371 (30.5, -10.5566) -> (28, -9.1132)
  line L372 (30.5, -13.4434) -> (30.5, -10.5566)
  line L373 (28, -14.8868) -> (30.5, -13.4434)
  line L374 (25.5, -13.4434) -> (28, -14.8868)
  line L375 (25.5, -10.5566) -> (25.5, -13.4434)
  line L376 (28, -9.1132) -> (25.5, -10.5566)
  line L377 (24.5, -8.8246) -> (27, -7.3812)
  line L378 (27, -7.3812) -> (27, -4.4944)
  line L379 (27, -4.4944) -> (24.5, -3.0511)
  line L380 (22, -7.3812) -> (24.5, -8.8246)
  line L381 (24.5, -3.0511) -> (22, -4.4944)
  line L382 (22, -4.4944) -> (22, -7.3812)
  line L383 (21, -9.1132) -> (18.5, -10.5566)
  line L384 (23.5, -10.5566) -> (21, -9.1132)
  line L385 (23.5, -13.4434) -> (23.5, -10.5566)
  line L386 (21, -14.8868) -> (23.5, -13.4434)
  line L387 (18.5, -13.4434) -> (21, -14.8868)
  line L388 (18.5, -10.5566) -> (18.5, -13.4434)
  line L389 (-24.5, 3.1754) -> (-22, 4.6188)
  line L390 (-22, 4.6188) -> (-22, 7.5056)
  line L391 (-22, 7.5056) -> (-24.5, 8.9489)
  line L392 (-24.5, 8.9489) -> (-27, 7.5056)
  line L393 (-27, 7.5056) -> (-27, 4.6188)
  line L394 (-27, 4.6188) -> (-24.5, 3.1754)
  line L395 (-25.5, 1.4434) -> (-28, 2.8868)
  line L396 (-25.5, -1.4434) -> (-25.5, 1.4434)
  line L397 (-28, -2.8868) -> (-25.5, -1.4434)
  line L398 (-30.5, -1.4434) -> (-28, -2.8868)
  line L399 (-30.5, 1.4434) -> (-30.5, -1.4434)
  line L400 (-28, 2.8868) -> (-30.5, 1.4434)
  line L401 (-31.5, 3.1754) -> (-29, 4.6188)
  line L402 (-29, 4.6188) -> (-29, 7.5056)
  line L403 (-29, 7.5056) -> (-31.5, 8.9489)
  line L404 (-34, 4.6188) -> (-31.5, 3.1754)
  line L405 (-31.5, 8.9489) -> (-34, 7.5056)
  line L406 (-34, 7.5056) -> (-34, 4.6188)
  line L407 (-35, 2.8868) -> (-37.5, 1.4434)
  line L408 (-32.5, 1.4434) -> (-35, 2.8868)
  line L409 (-32.5, -1.4434) -> (-32.5, 1.4434)
  line L410 (-35, -2.8868) -> (-32.5, -1.4434)
  line L411 (-37.5, -1.4434) -> (-35, -2.8868)
  line L412 (-37.5, 1.4434) -> (-37.5, -1.4434)
  line L413 (-10.5, 3.1754) -> (-8, 4.6188)
  line L414 (-8, 4.6188) -> (-8, 7.5056)
  line L415 (-8, 7.5056) -> (-10.5, 8.9489)
  line L416 (-10.5, 8.9489) -> (-13, 7.5056)
  line L417 (-13, 7.5056) -> (-13, 4.6188)
  line L418 (-13, 4.6188) -> (-10.5, 3.1754)
  line L419 (-11.5, 1.4434) -> (-14, 2.8868)
  line L420 (-11.5, -1.4434) -> (-11.5, 1.4434)
  line L421 (-14, -2.8868) -> (-11.5, -1.4434)
  line L422 (-16.5, -1.4434) -> (-14, -2.8868)
  line L423 (-16.5, 1.4434) -> (-16.5, -1.4434)
  line L424 (-14, 2.8868) -> (-16.5, 1.4434)
  line L425 (-17.5, 3.1754) -> (-15, 4.6188)
  line L426 (-15, 4.6188) -> (-15, 7.5056)
  line L427 (-15, 7.5056) -> (-17.5, 8.9489)
  line L428 (-20, 4.6188) -> (-17.5, 3.1754)
  line L429 (-17.5, 8.9489) -> (-20, 7.5056)
  line L430 (-20, 7.5056) -> (-20, 4.6188)
  line L431 (-21, 2.8868) -> (-23.5, 1.4434)
  line L432 (-18.5, 1.4434) -> (-21, 2.8868)
  line L433 (-18.5, -1.4434) -> (-18.5, 1.4434)
  line L434 (-21, -2.8868) -> (-18.5, -1.4434)
  line L435 (-23.5, -1.4434) -> (-21, -2.8868)
  line L436 (-23.5, 1.4434) -> (-23.5, -1.4434)
  line L437 (17.5, 3.1754) -> (20, 4.6188)
  line L438 (20, 4.6188) -> (20, 7.5056)
  line L439 (20, 7.5056) -> (17.5, 8.9489)
  line L440 (17.5, 8.9489) -> (15, 7.5056)
  line L441 (15, 7.5056) -> (15, 4.6188)
  line L442 (15, 4.6188) -> (17.5, 3.1754)
  line L443 (16.5, 1.4434) -> (14, 2.8868)
  line L444 (16.5, -1.4434) -> (16.5, 1.4434)
  line L445 (14, -2.8868) -> (16.5, -1.4434)
  line L446 (11.5, -1.4434) -> (14, -2.8868)
  line L447 (11.5, 1.4434) -> (11.5, -1.4434)
  line L448 (14, 2.8868) -> (11.5, 1.4434)
  line L449 (10.5, 3.1754) -> (13, 4.6188)
  line L450 (13, 4.6188) -> (13, 7.5056)
  line L451 (13, 7.5056) -> (10.5, 8.9489)
  line L452 (8, 4.6188) -> (10.5, 3.1754)
  line L453 (10.5, 8.9489) -> (8, 7.5056)
  line L454 (8, 7.5056) -> (8, 4.6188)
  line L455 (7, 2.8868) -> (4.5, 1.4434)
  line L456 (9.5, 1.4434) -> (7, 2.8868)
  line L457 (9.5, -1.4434) -> (9.5, 1.4434)
  line L458 (7, -2.8868) -> (9.5, -1.4434)
  line L459 (4.5, -1.4434) -> (7, -2.8868)
  line L460 (4.5, 1.4434) -> (4.5, -1.4434)
  line L461 (31.5, 3.1754) -> (34, 4.6188)
  line L462 (34, 4.6188) -> (34, 7.5056)
  line L463 (34, 7.5056) -> (31.5, 8.9489)
  line L464 (31.5, 8.9489) -> (29, 7.5056)
  line L465 (29, 7.5056) -> (29, 4.6188)
  line L466 (29, 4.6188) -> (31.5, 3.1754)
  line L467 (30.5, 1.4434) -> (28, 2.8868)
  line L468 (30.5, -1.4434) -> (30.5, 1.4434)
  line L469 (28, -2.8868) -> (30.5, -1.4434)
  line L470 (25.5, -1.4434) -> (28, -2.8868)
  line L471 (25.5, 1.4434) -> (25.5, -1.4434)
  line L472 (28, 2.8868) -> (25.5, 1.4434)
  line L473 (24.5, 3.1754) -> (27, 4.6188)
  line L474 (27, 4.6188) -> (27, 7.5056)
  line L475 (27, 7.5056) -> (24.5, 8.9489)
  line L476 (22, 4.6188) -> (24.5, 3.1754)
  line L477 (24.5, 8.9489) -> (22, 7.5056)
  line L478 (22, 7.5056) -> (22, 4.6188)
  line L479 (21, 2.8868) -> (18.5, 1.4434)
  line L480 (23.5, 1.4434) -> (21, 2.8868)
  line L481 (23.5, -1.4434) -> (23.5, 1.4434)
  line L482 (21, -2.8868) -> (23.5, -1.4434)
  line L483 (18.5, -1.4434) -> (21, -2.8868)
  line L484 (18.5, 1.4434) -> (18.5, -1.4434)
  line L485 (-24.5, 15.1754) -> (-22, 16.6188)
  line L486 (-22, 16.6188) -> (-22, 19.5056)
  line L487 (-22, 19.5056) -> (-24.5, 20.9489)
  line L488 (-24.5, 20.9489) -> (-27, 19.5056)
  line L489 (-27, 19.5056) -> (-27, 16.6188)
  line L490 (-27, 16.6188) -> (-24.5, 15.1754)
  line L491 (-25.5, 13.4434) -> (-28, 14.8868)
  line L492 (-25.5, 10.5566) -> (-25.5, 13.4434)
  line L493 (-28, 9.1132) -> (-25.5, 10.5566)
  line L494 (-30.5, 10.5566) -> (-28, 9.1132)
  line L495 (-30.5, 13.4434) -> (-30.5, 10.5566)
  line L496 (-28, 14.8868) -> (-30.5, 13.4434)
  line L497 (-31.5, 15.1754) -> (-29, 16.6188)
  line L498 (-29, 16.6188) -> (-29, 19.5056)
  line L499 (-29, 19.5056) -> (-31.5, 20.9489)
  line L500 (-34, 16.6188) -> (-31.5, 15.1754)
  line L501 (-31.5, 20.9489) -> (-34, 19.5056)
  line L502 (-34, 19.5056) -> (-34, 16.6188)
  line L503 (-35, 14.8868) -> (-37.5, 13.4434)
  line L504 (-32.5, 13.4434) -> (-35, 14.8868)
  line L505 (-32.5, 10.5566) -> (-32.5, 13.4434)
  line L506 (-35, 9.1132) -> (-32.5, 10.5566)
  line L507 (-37.5, 10.5566) -> (-35, 9.1132)
  line L508 (-37.5, 13.4434) -> (-37.5, 10.5566)
  line L509 (-10.5, 15.1754) -> (-8, 16.6188)
  line L510 (-8, 16.6188) -> (-8, 19.5056)
  line L511 (-8, 19.5056) -> (-10.5, 20.9489)
  line L512 (-10.5, 20.9489) -> (-13, 19.5056)
  line L513 (-13, 19.5056) -> (-13, 16.6188)
  line L514 (-13, 16.6188) -> (-10.5, 15.1754)
  line L515 (-11.5, 13.4434) -> (-14, 14.8868)
  line L516 (-11.5, 10.5566) -> (-11.5, 13.4434)
  line L517 (-14, 9.1132) -> (-11.5, 10.5566)
  line L518 (-16.5, 10.5566) -> (-14, 9.1132)
  line L519 (-16.5, 13.4434) -> (-16.5, 10.5566)
  line L520 (-14, 14.8868) -> (-16.5, 13.4434)
  line L521 (-17.5, 15.1754) -> (-15, 16.6188)
  line L522 (-15, 16.6188) -> (-15, 19.5056)
  line L523 (-15, 19.5056) -> (-17.5, 20.9489)
  line L524 (-20, 16.6188) -> (-17.5, 15.1754)
  line L525 (-17.5, 20.9489) -> (-20, 19.5056)
  line L526 (-20, 19.5056) -> (-20, 16.6188)
  line L527 (-21, 14.8868) -> (-23.5, 13.4434)
  line L528 (-18.5, 13.4434) -> (-21, 14.8868)
  line L529 (-18.5, 10.5566) -> (-18.5, 13.4434)
  line L530 (-21, 9.1132) -> (-18.5, 10.5566)
  line L531 (-23.5, 10.5566) -> (-21, 9.1132)
  line L532 (-23.5, 13.4434) -> (-23.5, 10.5566)
  line L533 (3.5, 15.1754) -> (6, 16.6188)
  line L534 (6, 16.6188) -> (6, 19.5056)
  line L535 (6, 19.5056) -> (3.5, 20.9489)
  line L536 (3.5, 20.9489) -> (1, 19.5056)
  line L537 (1, 19.5056) -> (1, 16.6188)
  line L538 (1, 16.6188) -> (3.5, 15.1754)
  line L539 (2.5, 13.4434) -> (0, 14.8868)
  line L540 (2.5, 10.5566) -> (2.5, 13.4434)
  line L541 (0, 9.1132) -> (2.5, 10.5566)
  line L542 (-2.5, 10.5566) -> (0, 9.1132)
  line L543 (-2.5, 13.4434) -> (-2.5, 10.5566)
  line L544 (0, 14.8868) -> (-2.5, 13.4434)
  line L545 (-3.5, 15.1754) -> (-1, 16.6188)
  line L546 (-1, 16.6188) -> (-1, 19.5056)
  line L547 (-1, 19.5056) -> (-3.5, 20.9489)
  line L548 (-6, 16.6188) -> (-3.5, 15.1754)
  line L549 (-3.5, 20.9489) -> (-6, 19.5056)
  line L550 (-6, 19.5056) -> (-6, 16.6188)
  line L551 (-7, 14.8868) -> (-9.5, 13.4434)
  line L552 (-4.5, 13.4434) -> (-7, 14.8868)
  line L553 (-4.5, 10.5566) -> (-4.5, 13.4434)
  line L554 (-7, 9.1132) -> (-4.5, 10.5566)
  line L555 (-9.5, 10.5566) -> (-7, 9.1132)
  line L556 (-9.5, 13.4434) -> (-9.5, 10.5566)
  line L557 (17.5, 15.1754) -> (20, 16.6188)
  line L558 (20, 16.6188) -> (20, 19.5056)
  line L559 (20, 19.5056) -> (17.5, 20.9489)
  line L560 (17.5, 20.9489) -> (15, 19.5056)
  line L561 (15, 19.5056) -> (15, 16.6188)
  line L562 (15, 16.6188) -> (17.5, 15.1754)
  line L563 (16.5, 13.4434) -> (14, 14.8868)
  line L564 (16.5, 10.5566) -> (16.5, 13.4434)
  line L565 (14, 9.1132) -> (16.5, 10.5566)
  line L566 (11.5, 10.5566) -> (14, 9.1132)
  line L567 (11.5, 13.4434) -> (11.5, 10.5566)
  line L568 (14, 14.8868) -> (11.5, 13.4434)
  line L569 (10.5, 15.1754) -> (13, 16.6188)
  line L570 (13, 16.6188) -> (13, 19.5056)
  line L571 (13, 19.5056) -> (10.5, 20.9489)
  line L572 (8, 16.6188) -> (10.5, 15.1754)
  line L573 (10.5, 20.9489) -> (8, 19.5056)
  line L574 (8, 19.5056) -> (8, 16.6188)
  line L575 (7, 14.8868) -> (4.5, 13.4434)
  line L576 (9.5, 13.4434) -> (7, 14.8868)
  line L577 (9.5, 10.5566) -> (9.5, 13.4434)
  line L578 (7, 9.1132) -> (9.5, 10.5566)
  line L579 (4.5, 10.5566) -> (7, 9.1132)
  line L580 (4.5, 13.4434) -> (4.5, 10.5566)
  line L581 (31.5, 15.1754) -> (34, 16.6188)
  line L582 (34, 16.6188) -> (34, 19.5056)
  line L583 (34, 19.5056) -> (31.5, 20.9489)
  line L584 (31.5, 20.9489) -> (29, 19.5056)
  line L585 (29, 19.5056) -> (29, 16.6188)
  line L586 (29, 16.6188) -> (31.5, 15.1754)
  line L587 (30.5, 13.4434) -> (28, 14.8868)
  line L588 (30.5, 10.5566) -> (30.5, 13.4434)
  line L589 (28, 9.1132) -> (30.5, 10.5566)
  line L590 (25.5, 10.5566) -> (28, 9.1132)
  line L591 (25.5, 13.4434) -> (25.5, 10.5566)
  line L592 (28, 14.8868) -> (25.5, 13.4434)
  line L593 (24.5, 15.1754) -> (27, 16.6188)
  line L594 (27, 16.6188) -> (27, 19.5056)
  line L595 (27, 19.5056) -> (24.5, 20.9489)
  line L596 (22, 16.6188) -> (24.5, 15.1754)
  line L597 (24.5, 20.9489) -> (22, 19.5056)
  line L598 (22, 19.5056) -> (22, 16.6188)
  line L599 (21, 14.8868) -> (18.5, 13.4434)
  line L600 (23.5, 13.4434) -> (21, 14.8868)
  line L601 (23.5, 10.5566) -> (23.5, 13.4434)
  line L602 (21, 9.1132) -> (23.5, 10.5566)
  line L603 (18.5, 10.5566) -> (21, 9.1132)
  line L604 (18.5, 13.4434) -> (18.5, 10.5566)
  line L605 (-24.5, 27.1754) -> (-22, 28.6188)
  line L606 (-22, 28.6188) -> (-22, 31.5056)
  line L607 (-22, 31.5056) -> (-24.5, 32.9489)
  line L608 (-24.5, 32.9489) -> (-27, 31.5056)
  line L609 (-27, 31.5056) -> (-27, 28.6188)
  line L610 (-27, 28.6188) -> (-24.5, 27.1754)
  line L611 (-25.5, 25.4434) -> (-28, 26.8868)
  line L612 (-25.5, 22.5566) -> (-25.5, 25.4434)
  line L613 (-28, 21.1132) -> (-25.5, 22.5566)
  line L614 (-30.5, 22.5566) -> (-28, 21.1132)
  line L615 (-30.5, 25.4434) -> (-30.5, 22.5566)
  line L616 (-28, 26.8868) -> (-30.5, 25.4434)
  line L617 (-31.5, 27.1754) -> (-29, 28.6188)
  line L618 (-29, 28.6188) -> (-29, 31.5056)
  line L619 (-29, 31.5056) -> (-31.5, 32.9489)
  line L620 (-34, 28.6188) -> (-31.5, 27.1754)
  line L621 (-31.5, 32.9489) -> (-34, 31.5056)
  line L622 (-34, 31.5056) -> (-34, 28.6188)
  line L623 (-35, 26.8868) -> (-37.5, 25.4434)
  line L624 (-32.5, 25.4434) -> (-35, 26.8868)
  line L625 (-32.5, 22.5566) -> (-32.5, 25.4434)
  line L626 (-35, 21.1132) -> (-32.5, 22.5566)
  line L627 (-37.5, 22.5566) -> (-35, 21.1132)
  line L628 (-37.5, 25.4434) -> (-37.5, 22.5566)
  line L629 (-10.5, 27.1754) -> (-8, 28.6188)
  line L630 (-8, 28.6188) -> (-8, 31.5056)
  line L631 (-8, 31.5056) -> (-10.5, 32.9489)
  line L632 (-10.5, 32.9489) -> (-13, 31.5056)
  line L633 (-13, 31.5056) -> (-13, 28.6188)
  line L634 (-13, 28.6188) -> (-10.5, 27.1754)
  line L635 (-11.5, 25.4434) -> (-14, 26.8868)
  line L636 (-11.5, 22.5566) -> (-11.5, 25.4434)
  line L637 (-14, 21.1132) -> (-11.5, 22.5566)
  line L638 (-16.5, 22.5566) -> (-14, 21.1132)
  line L639 (-16.5, 25.4434) -> (-16.5, 22.5566)
  line L640 (-14, 26.8868) -> (-16.5, 25.4434)
  line L641 (-17.5, 27.1754) -> (-15, 28.6188)
  line L642 (-15, 28.6188) -> (-15, 31.5056)
  line L643 (-15, 31.5056) -> (-17.5, 32.9489)
  line L644 (-20, 28.6188) -> (-17.5, 27.1754)
  line L645 (-17.5, 32.9489) -> (-20, 31.5056)
  line L646 (-20, 31.5056) -> (-20, 28.6188)
  line L647 (-21, 26.8868) -> (-23.5, 25.4434)
  line L648 (-18.5, 25.4434) -> (-21, 26.8868)
  line L649 (-18.5, 22.5566) -> (-18.5, 25.4434)
  line L650 (-21, 21.1132) -> (-18.5, 22.5566)
  line L651 (-23.5, 22.5566) -> (-21, 21.1132)
  line L652 (-23.5, 25.4434) -> (-23.5, 22.5566)
  line L653 (3.5, 27.1754) -> (6, 28.6188)
  line L654 (6, 28.6188) -> (6, 31.5056)
  line L655 (6, 31.5056) -> (3.5, 32.9489)
  line L656 (3.5, 32.9489) -> (1, 31.5056)
  line L657 (1, 31.5056) -> (1, 28.6188)
  line L658 (1, 28.6188) -> (3.5, 27.1754)
  line L659 (2.5, 25.4434) -> (0, 26.8868)
  line L660 (2.5, 22.5566) -> (2.5, 25.4434)
  line L661 (0, 21.1132) -> (2.5, 22.5566)
  line L662 (-2.5, 22.5566) -> (0, 21.1132)
  line L663 (-2.5, 25.4434) -> (-2.5, 22.5566)
  line L664 (0, 26.8868) -> (-2.5, 25.4434)
  line L665 (-3.5, 27.1754) -> (-1, 28.6188)
  line L666 (-1, 28.6188) -> (-1, 31.5056)
  line L667 (-1, 31.5056) -> (-3.5, 32.9489)
  line L668 (-6, 28.6188) -> (-3.5, 27.1754)
  line L669 (-3.5, 32.9489) -> (-6, 31.5056)
  line L670 (-6, 31.5056) -> (-6, 28.6188)
  line L671 (-7, 26.8868) -> (-9.5, 25.4434)
  line L672 (-4.5, 25.4434) -> (-7, 26.8868)
  line L673 (-4.5, 22.5566) -> (-4.5, 25.4434)
  line L674 (-7, 21.1132) -> (-4.5, 22.5566)
  line L675 (-9.5, 22.5566) -> (-7, 21.1132)
  line L676 (-9.5, 25.4434) -> (-9.5, 22.5566)
  line L677 (17.5, 27.1754) -> (20, 28.6188)
  line L678 (20, 28.6188) -> (20, 31.5056)
  line L679 (20, 31.5056) -> (17.5, 32.9489)
  line L680 (17.5, 32.9489) -> (15, 31.5056)
  line L681 (15, 31.5056) -> (15, 28.6188)
  line L682 (15, 28.6188) -> (17.5, 27.1754)
  line L683 (16.5, 25.4434) -> (14, 26.8868)
  line L684 (16.5, 22.5566) -> (16.5, 25.4434)
  line L685 (14, 21.1132) -> (16.5, 22.5566)
  line L686 (11.5, 22.5566) -> (14, 21.1132)
  line L687 (11.5, 25.4434) -> (11.5, 22.5566)
  line L688 (14, 26.8868) -> (11.5, 25.4434)
  line L689 (10.5, 27.1754) -> (13, 28.6188)
  line L690 (13, 28.6188) -> (13, 31.5056)
  line L691 (13, 31.5056) -> (10.5, 32.9489)
  line L692 (8, 28.6188) -> (10.5, 27.1754)
  line L693 (10.5, 32.9489) -> (8, 31.5056)
  line L694 (8, 31.5056) -> (8, 28.6188)
  line L695 (7, 26.8868) -> (4.5, 25.4434)
  line L696 (9.5, 25.4434) -> (7, 26.8868)
  line L697 (9.5, 22.5566) -> (9.5, 25.4434)
  line L698 (7, 21.1132) -> (9.5, 22.5566)
  line L699 (4.5, 22.5566) -> (7, 21.1132)
  line L700 (4.5, 25.4434) -> (4.5, 22.5566)
  line L701 (31.5, 27.1754) -> (34, 28.6188)
  line L702 (34, 28.6188) -> (34, 31.5056)
  line L703 (34, 31.5056) -> (31.5, 32.9489)
  line L704 (31.5, 32.9489) -> (29, 31.5056)
  line L705 (29, 31.5056) -> (29, 28.6188)
  line L706 (29, 28.6188) -> (31.5, 27.1754)
  line L707 (30.5, 25.4434) -> (28, 26.8868)
  line L708 (30.5, 22.5566) -> (30.5, 25.4434)
  line L709 (28, 21.1132) -> (30.5, 22.5566)
  line L710 (25.5, 22.5566) -> (28, 21.1132)
  line L711 (25.5, 25.4434) -> (25.5, 22.5566)
  line L712 (28, 26.8868) -> (25.5, 25.4434)
  line L713 (24.5, 27.1754) -> (27, 28.6188)
  line L714 (27, 28.6188) -> (27, 31.5056)
  line L715 (27, 31.5056) -> (24.5, 32.9489)
  line L716 (22, 28.6188) -> (24.5, 27.1754)
  line L717 (24.5, 32.9489) -> (22, 31.5056)
  line L718 (22, 31.5056) -> (22, 28.6188)
  line L719 (21, 26.8868) -> (18.5, 25.4434)
  line L720 (23.5, 25.4434) -> (21, 26.8868)
  line L721 (23.5, 22.5566) -> (23.5, 25.4434)
  line L722 (21, 21.1132) -> (23.5, 22.5566)
  line L723 (18.5, 22.5566) -> (21, 21.1132)
  line L724 (18.5, 25.4434) -> (18.5, 22.5566)
  line L725 (-24.5, 39.1754) -> (-22, 40.6188)
  line L726 (-22, 40.6188) -> (-22, 43.5056)
  line L727 (-22, 43.5056) -> (-24.5, 44.9489)
  line L728 (-24.5, 44.9489) -> (-27, 43.5056)
  line L729 (-27, 43.5056) -> (-27, 40.6188)
  line L730 (-27, 40.6188) -> (-24.5, 39.1754)
  line L731 (-25.5, 37.4434) -> (-28, 38.8868)
  line L732 (-25.5, 34.5566) -> (-25.5, 37.4434)
  line L733 (-28, 33.1132) -> (-25.5, 34.5566)
  line L734 (-30.5, 34.5566) -> (-28, 33.1132)
  line L735 (-30.5, 37.4434) -> (-30.5, 34.5566)
  line L736 (-28, 38.8868) -> (-30.5, 37.4434)
  line L737 (-31.5, 39.1754) -> (-29, 40.6188)
  line L738 (-29, 40.6188) -> (-29, 43.5056)
  line L739 (-29, 43.5056) -> (-31.5, 44.9489)
  line L740 (-34, 40.6188) -> (-31.5, 39.1754)
  line L741 (-31.5, 44.9489) -> (-34, 43.5056)
  line L742 (-34, 43.5056) -> (-34, 40.6188)
  line L743 (-35, 38.8868) -> (-37.5, 37.4434)
  line L744 (-32.5, 37.4434) -> (-35, 38.8868)
  line L745 (-32.5, 34.5566) -> (-32.5, 37.4434)
  line L746 (-35, 33.1132) -> (-32.5, 34.5566)
  line L747 (-37.5, 34.5566) -> (-35, 33.1132)
  line L748 (-37.5, 37.4434) -> (-37.5, 34.5566)
  line L749 (-10.5, 39.1754) -> (-8, 40.6188)
  line L750 (-8, 40.6188) -> (-8, 43.5056)
  line L751 (-8, 43.5056) -> (-10.5, 44.9489)
  line L752 (-10.5, 44.9489) -> (-13, 43.5056)
  line L753 (-13, 43.5056) -> (-13, 40.6188)
  line L754 (-13, 40.6188) -> (-10.5, 39.1754)
  line L755 (-11.5, 37.4434) -> (-14, 38.8868)
  line L756 (-11.5, 34.5566) -> (-11.5, 37.4434)
  line L757 (-14, 33.1132) -> (-11.5, 34.5566)
  line L758 (-16.5, 34.5566) -> (-14, 33.1132)
  line L759 (-16.5, 37.4434) -> (-16.5, 34.5566)
  line L760 (-14, 38.8868) -> (-16.5, 37.4434)
  line L761 (-17.5, 39.1754) -> (-15, 40.6188)
  line L762 (-15, 40.6188) -> (-15, 43.5056)
  line L763 (-15, 43.5056) -> (-17.5, 44.9489)
  line L764 (-20, 40.6188) -> (-17.5, 39.1754)
  line L765 (-17.5, 44.9489) -> (-20, 43.5056)
  line L766 (-20, 43.5056) -> (-20, 40.6188)
  line L767 (-21, 38.8868) -> (-23.5, 37.4434)
  line L768 (-18.5, 37.4434) -> (-21, 38.8868)